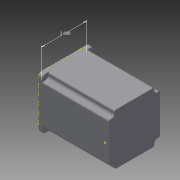
# Autodesk Inventor part: G723-280-4
Saved by Autodesk Inventor 2013 (Build 170138000, 138)
## iProperties
Created: 2012-11-28
Part Number: G723-280-4
Material: Generic
Document SubType Name: Modeling
Designer: istvan.burbank
Density: 1 g/cm^3
Mass: 258.816 g
Surface Area: 246.452 cm^2
Volume: 258.816 cm^3
Author: istvan.burbank
Autodesk Inventor part; units mm, degrees
ref_plane "YZ Plane" through (0, 0, 0) normal (1, 0, 0) x (0, 1, 0)
ref_plane "XZ Plane" through (0, 0, 0) normal (0, 1, 0) x (-1, 0, 0)
ref_plane "XY Plane" through (0, 0, 0) normal (0, 0, 1) x (1, 0, 0)
sketch "Sketch1" plane through (0, 0, 0) normal (1, 0, 0) x (0, 1, 0)
  line L0 (3.175, 0) -> (53.975, 0)
  line L1 (57.15, 3.175) -> (57.15, 53.975)
  line L2 (53.975, 57.15) -> (3.175, 57.15)
  line L3 (0, 53.975) -> (0, 3.175)
  arc A0 (3.175, 57.15) -> (0, 53.975) centre (3.175, 53.975) ccw
  arc A1 (57.15, 53.975) -> (53.975, 57.15) centre (53.975, 53.975) ccw
  arc A2 (53.975, 0) -> (57.15, 3.175) centre (53.975, 3.175) ccw
  arc A3 (0, 3.175) -> (3.175, 0) centre (3.175, 3.175) ccw
  point P0 (0, 0)
  point P1 (57.15, 57.15)
  point P2 (57.15, 0)
  point P3 (0, 57.15)
  dimension "d0" = 57.15
  dimension "d1" = 57.15
  dimension "d17" = 3.175
  constraints: 8 end point, 8 point on circle, 8 point on line, 8 tangent, 4 centre point, 3 equal radius, 2 parallel, 1 horizontal, 1 perpendicular
  measures "d0" distance of point (0, 57.15) point (57.15, 57.15)
  measures "d1" distance of point (57.15, 57.15) point (57.15, 0)
  measures "d17" radius of A0
extrude "Extrusion1" add sketch "Sketch1" along normal blind 78.74
sketch "Sketch2" plane through (0, 0, 0) normal (-1, 0, 0) x (0, 0, 1)
  line L0 (0, 53.975) -> (0, 3.175) projected
  line L1 (53.975, 57.15) -> (3.175, 57.15) projected
  circle A0 centre (28.575, 28.575) radius 19.05
  point P0 (0, 57.15)
  point P1 (0, 0)
  point P2 (57.15, 57.15)
  dimension "d4" = 38.1
  dimension "d18" = 28.575
  dimension "d19" = 28.575
  constraints: 1 centre point
  measures "d4" diameter of A0
  measures "d18" distance from line of L1 A0.centre
  measures "d19" distance from line of L0 A0.centre
extrude "Extrusion2" add sketch "Sketch2" along normal blind 1.524
sketch "Sketch3" plane through (-1.524, 28.575, 28.575) normal (-1, 0, 0) x (0, 0, 1)
  circle A0 centre (0, 0) radius 19.05 projected
  circle A1 centre (0, 0) radius 3.175
  point P0 (-28.575, -28.575)
  dimension "d10" = 6.35
  constraints: 1 centre point, 1 coincident
  measures "d10" diameter of A1
extrude "Extrusion3" add sketch "Sketch3" along normal blind 19.05 contours A1
sketch "Sketch4" plane through (-20.574, 28.575, 28.575) normal (-1, 0, 0) x (0, 0, 1)
  circle A0 centre (0, 0) radius 3.175 projected
  line L0 (-1.7227, 2.667) -> (1.7227, 2.667)
  line L1 (0, -3.175) -> (-5.2914, -3.175)
  point P0 (-28.575, -28.575)
  dimension "d13" = 5.842
  constraints: 4 end point, 3 point on circle, 1 horizontal, 1 parallel, 1 tangent
  measures "d13" distance between parallel lines of L0 L1
extrude "Extrusion4" cut sketch "Sketch4" against normal blind 14.986 contours L0 A0 picked at (-0.1211, 2.8294)
sketch "Sketch5" plane through (78.74, 0, 0) normal (1, 0, 0) x (0, 0, -1)
  arc A0 (-57.15, 3.175) -> (-53.975, 0) centre (-53.975, 3.175) ccw projected
  arc A1 (-3.175, 0) -> (0, 3.175) centre (-3.175, 3.175) ccw projected
  arc A2 (0, 53.975) -> (-3.175, 57.15) centre (-3.175, 53.975) ccw projected
  arc A3 (-53.975, 57.15) -> (-57.15, 53.975) centre (-53.975, 53.975) ccw projected
  circle A4 centre (-53.975, 53.975) radius 3.175
  circle A5 centre (-3.175, 53.975) radius 3.175
  circle A6 centre (-3.175, 3.175) radius 3.175
  circle A7 centre (-53.975, 3.175) radius 3.175
  line L0 (-57.15, 53.975) -> (-57.15, 3.175) projected
  line L1 (-53.975, 0) -> (-3.175, 0) projected
  line L2 (0, 3.175) -> (0, 53.975) projected
  line L3 (-3.175, 57.15) -> (-53.975, 57.15) projected
  line L4 (-6.35, 57.15) -> (0, 57.15)
  line L5 (0, 57.15) -> (0, 50.8)
  line L6 (0, 50.8) -> (-3.175, 50.8)
  line L7 (-6.35, 53.975) -> (-6.35, 57.15)
  line L8 (-50.8, 57.15) -> (-57.15, 57.15)
  line L9 (-57.15, 57.15) -> (-57.15, 50.8)
  line L10 (-57.15, 50.8) -> (-53.975, 50.8)
  line L11 (-50.8, 53.975) -> (-50.8, 57.15)
  line L12 (-57.15, 6.35) -> (-53.975, 6.35)
  line L13 (-50.8, 3.175) -> (-50.8, 0)
  line L14 (-50.8, 0) -> (-57.15, 0)
  line L15 (-57.15, 0) -> (-57.15, 6.35)
  line L16 (-6.35, 0) -> (0, 0)
  line L17 (0, 0) -> (0, 6.35)
  line L18 (0, 6.35) -> (-3.175, 6.35)
  line L19 (-6.35, 3.175) -> (-6.35, 0)
  point P0 (0, 0)
  dimension "d22" = 6.35
  dimension "d24" = 6.35
  dimension "d25" = 6.35
  dimension "d26" = 6.35
  dimension "d27" = 6.35
  dimension "d28" = 6.35
  dimension "d29" = 6.35
  dimension "d30" = 6.35
  dimension "d31" = 6.35
  dimension "d32" = 6.35
  constraints: 32 end point, 8 parallel, 8 point on circle, 8 point on line, 4 centre point, 4 coincident, 4 horizontal, 4 perpendicular, 2 concentric
  measures "d22" diameter of A5
  measures "d24" diameter of A7
  measures "d25" distance between parallel lines of L9 L11
  measures "d26" distance between parallel lines of L10 L8
  measures "d27" distance between parallel lines of L5 L7
  measures "d28" distance between parallel lines of L6 L4
  measures "d29" distance between parallel lines of L1 L12
  measures "d30" distance between parallel lines of L13 L0
  measures "d31" distance between parallel lines of L16 L18
  measures "d32" distance between parallel lines of L2 L19
extrude "Extrusion6" cut sketch "Sketch5" against normal blind 74.041 contours A7 A0 | L0 L12 A7 | A0 L14 L15 | A7 L13 L1 | L0 A4 L10 | L19 A6 L1 | L9 L8 A3 | A3 A4 | A6 A1 | A1 L17 L16 | L3 L11 A4 | A6 L18 L2 | L3 A5 L7 | L6 A5 L2 | L4 L5 A2 | A2 A5
fillet "Fillet1" radius 1.905 8 edges at (41.7195, 57.15, 50.8) (41.7195, 50.8, 57.15) (41.7195, 57.15, 6.35) (41.7195, 50.8, 0) (41.7195, 6.35, 57.15) (41.7195, 0, 50.8) (41.7195, 6.35, 0) (41.7195, 0, 6.35)
sketch "Sketch6" plane through (0, 0, 0) normal (-1, 0, 0) x (0, 0, 1)
  circle A0 centre (28.575, 28.575) radius 19.05 projected
  line L0 (57.15, 3.175) -> (57.15, 53.975) projected
  arc A1 (57.15, 53.975) -> (53.975, 57.15) centre (53.975, 53.975) ccw projected
  line L1 (53.975, 57.15) -> (3.175, 57.15) projected
  arc A2 (3.175, 57.15) -> (0, 53.975) centre (3.175, 53.975) ccw projected
  line L2 (0, 53.975) -> (0, 3.175) projected
  arc A3 (0, 3.175) -> (3.175, 0) centre (3.175, 3.175) ccw projected
  line L3 (3.175, 0) -> (53.975, 0) projected
  arc A4 (53.975, 0) -> (57.15, 3.175) centre (53.975, 3.175) ccw projected
  point P0 (0, 0)
  point P1 (3.175, 49.6925)
  point P2 (53.975, 48.7357)
  point P3 (52.6312, 9.525)
  point P4 (6.4324, 8.0042)
  dimension "d36" = 50.8
  measures "d36" horizontal distance of point (53.975, 48.736) point (3.175, 49.693)
body "Solid1"
